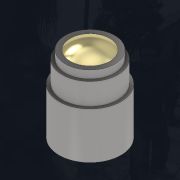
# Autodesk Inventor part: button 3
Saved by Autodesk Inventor 2021 (Build 250183000, 183)
## iProperties
Created: 2021-01-12
Part Number: button 3
Material: Generic
Document SubType Name: Modeling
Designer: Alex
Density: 1 g/cm^3
Appearance: Default
Author: Alex
Autodesk Inventor part; units mm, degrees
ref_plane "YZ Plane" through (0, 0, 0) normal (1, 0, 0) x (0, 1, 0)
ref_plane "XZ Plane" through (0, 0, 0) normal (0, 1, 0) x (-1, 0, 0)
ref_plane "XY Plane" through (0, 0, 0) normal (0, 0, 1) x (1, 0, 0)
sketch "Sketch1" plane through (0, 0, 0) normal (0, 1, 0) x (-1, 0, 0)
  arc A0 (8, 6) -> (8, -6) centre (0, 0) ccw
  arc A1 (7, 5.6569) -> (7, -5.6569) centre (0, 0) ccw
  line L0 (8, 0) -> (8, -6)
  line L1 (8, 6) -> (8, 0)
  line L2 (7, -5.6569) -> (7, 5.6569)
  dimension "d0" = 20
  dimension "d1" = 1
  constraints: 6 end point, 4 point on circle, 2 centre point, 1 coincident, 1 collinear, 1 point on line, 1 vertical
  measures "d0" diameter of A0
  measures "d1" radial gap between concentric circles of A0 A1
extrude "Extrusion1" add sketch "Sketch1" along normal blind 8
sketch "Sketch2" plane through (0, 0, 0) normal (0, -1, 0) x (1, 0, 0)
  point P0 (0, 0)
sketch "Sketch3" plane through (-8, 0, -6) normal (-1, 0, 0) x (0, 0, 1)
  line L0 (0, 8) -> (12, 8) construction
  line L1 (6, 8) -> (6, -6) construction
  circle A0 centre (6, -6) radius 14
  point P0 (6, 0)
  dimension "d7" = 14
  constraints: 2 end point, 1 coincident, 1 midpoint, 1 vertical, 1 vertical alignment, 2 other
  measures "d7" distance of L1.start L1.end
sketch "Sketch4" plane through (0, 8, 0) normal (0, 1, 0) x (1, 0, 0)
  circle A0 centre (0, 0) radius 10
  circle A1 centre (0, 0) radius 9
  constraints: 2 centre point, 2 coincident
extrude "Extrusion2" add sketch "Sketch4" against normal blind 8
extrude "Extrusion3" cut sketch "Sketch3" along normal blind 8
sketch "Sketch5" plane through (0, 8, 0) normal (0, 1, 0) x (1, 0, 0)
  circle A0 centre (0, 0) radius 10
  circle A1 centre (0, 0) radius 9
  constraints: 2 centre point, 2 coincident
extrude "Extrusion4" add sketch "Sketch5" along normal blind 7
sketch "Sketch6" plane through (0, 15, 0) normal (0, 1, 0) x (1, 0, 0)
  circle A0 centre (0, 0) radius 9
  arc A1 (-7, -5.6569) -> (-7, 5.6569) centre (0, 0) ccw projected
  circle A2 centre (0, 0) radius 8
  dimension "d14" = 16
  constraints: 2 centre point, 2 coincident
  measures "d14" diameter of A2
extrude "Extrusion5" add sketch "Sketch6" against normal up to surface (7 mm away)
sketch "Sketch7" plane through (0, 8, 0) normal (0, -1, 0) x (1, 0, 0)
  arc A0 (-8, 4.1231) -> (-9, 0) centre (0, 0) ccw projected
  circle A1 centre (0, 0) radius 9
  circle A2 centre (0, 0) radius 8
  line L0 (-8, -4.1231) -> (-8, 0) projected
  line L1 (-8, 0) -> (-8, 4.1231) projected
  line L2 (-8, -4.1231) -> (-8, 4.1231)
  line L3 (-7, 5.6569) -> (-7, 3.873) projected
  line L4 (-7, -3.873) -> (-7, -5.6569) projected
  line L5 (-7, 5.6569) -> (-7, -5.6569)
  constraints: 4 end point, 2 centre point, 2 coincident, 2 collinear, 1 point on circle
extrude "Extrusion6" add sketch "Sketch7" along normal up to surface (8 mm away) contours A1 L4 A2 L3
sketch "Sketch8" plane through (0, 15, 0) normal (0, 1, 0) x (1, 0, 0)
  circle A0 centre (0, 0) radius 9
  circle A1 centre (0, 0) radius 8
  circle A2 centre (0, 0) radius 9
  dimension "d19" = 18
  constraints: 3 centre point, 3 coincident, 1 concentric
  measures "d19" diameter of A0
extrude "Extrusion7" add sketch "Sketch8" along normal blind 7
sketch "Sketch9" plane through (0, 22, 0) normal (0, 1, 0) x (1, 0, 0)
  circle A0 centre (0, 0) radius 8
  circle A1 centre (0, 0) radius 7
  dimension "d22" = 14
  constraints: 2 centre point, 2 coincident
  measures "d22" diameter of A1
extrude "Extrusion8" add sketch "Sketch9" against normal up to surface (22 mm away)
sketch "Sketch10" plane through (0, 22, 0) normal (0, 1, 0) x (1, 0, 0)
  circle A0 centre (0, 0) radius 7
  circle A1 centre (0, 0) radius 7 projected
  circle A2 centre (0, 0) radius 8
  dimension "d25" = 16
  constraints: 2 centre point, 2 coincident
  measures "d25" diameter of A2
extrude "Extrusion9" add sketch "Sketch10" along normal blind 2.5
sketch "Sketch11" plane through (0, 24.5, 0) normal (0, 1, 0) x (1, 0, 0)
  circle A0 centre (0, 0) radius 8
  circle A1 centre (0, 0) radius 7
  circle A2 centre (0, 0) radius 7
  constraints: 3 centre point, 3 coincident
extrude "Extrusion10" add sketch "Sketch11" against normal up to surface (24.5 mm away) contours A1
sketch "Sketch13" plane through (0, 0, 0) normal (0, 0, 1) x (1, 0, 0)
  line L0 (0, 24.5) -> (6.4, 24.5)
  line L1 (0, 24.5) -> (6.4, 24.5)
  line L2 (0, 26.5) -> (0, 24.5)
  arc A0 (6.4, 24.5) -> (0, 26.5) centre (0, 15.26) ccw
  line L3 (0, 0) -> (0, 24.5)
  line L4 (8, 24.5) -> (-8, 24.5) projected
  constraints: 8 end point, 2 midpoint, 2 point on circle, 1 centre point, 1 coincident, 1 vertical
revolve "Revolution1" add sketch "Sketch13" angle 360 about axis through (0, 26.5, 0) along (0, -1, 0)
body "Solid1"
